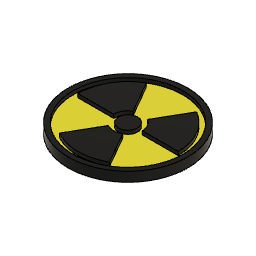
Radioactive_symbol (Autodesk Fusion 360 design; units mm, degrees)
Autodesk Fusion 360 part; units mm, degrees
sketch "Sketch2" plane through (0, 0, 0) normal (0, 0, 1) x (1, 0, 0)
  circle A0 centre (0, 0) radius 25
  dimension "d3" = 50
  constraint coincident A0.centre origin
  measures "d3" diameter of A0
extrude "Extrude2" add sketch "Sketch2" along normal blind 2.5
sketch "Sketch3" plane through (0, 0, 2.5) normal (0, 0, 1) x (-1, 0, 0)
  circle A0 centre (0, 0) radius 25
  circle A1 centre (0, 0) radius 23
  circle A2 centre (0, 0) radius 21
  circle A3 centre (0, 0) radius 4
  line L0 (6, 0) -> (3, 5.1962) construction
  line L1 (3, 5.1962) -> (-3, 5.1962) construction
  line L2 (-3, 5.1962) -> (-6, 0) construction
  line L3 (-6, 0) -> (-3, -5.1962) construction
  line L4 (-3, -5.1962) -> (3, -5.1962) construction
  line L5 (3, -5.1962) -> (6, 0) construction
  line L6 (-3, -5.1962) -> (-10.5, -18.1865)
  line L7 (-6, 0) -> (-21, 0)
  line L8 (-3, 5.1962) -> (-10.5, 18.1865)
  line L9 (3, 5.1962) -> (10.5, 18.1865)
  line L10 (6, 0) -> (21, 0)
  line L11 (3, -5.1962) -> (10.5, -18.1865)
  line L12 (21, 0) -> (10.5, -18.1865) construction
  line L13 (-10.5, -18.1865) -> (-21, 0) construction
  line L14 (-10.5, 18.1865) -> (-21, 0) construction
  line L15 (-10.5, -18.1865) -> (10.5, -18.1865) construction
  line L16 (21, 0) -> (10.5, 18.1865) construction
  circle A4 centre (0, 0) radius 6
  dimension "d6" = -2
  dimension "d7" = -4
  dimension "d8" = 8
  dimension "d9" = 6
  constraint coincident A0.centre A1.centre
  constraint horizontal L4
  constraint coincident A2 L6.end
  constraint coincident A2 L7.end
  constraint coincident A2 L8.end
  constraint coincident A2 L9.end
  constraint coincident A2 L10.end
  constraint parallel L7 L10
  constraint coincident A2 L11.end
  constraint equal L12 L16
  constraint equal L13 L15
  constraint equal L12 L15
  constraint equal L13 L14
  constraint horizontal L10
  constraint coincident L3.end A4
  measures "d8" diameter of A3
  measures "d9" distance of L0.start A0.centre
extrude "Extrude3" add sketch "Sketch3" along normal blind 1.5 contours A0 | A2 L10 L11 A4 | A2 L8 L9 A4 | A2 L6 L7 A4
extrude "Extrude4" add sketch "Sketch3" along normal blind 1.5 contours A3
